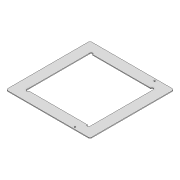
# Autodesk Inventor part: Limiter
Saved by Autodesk Inventor 2020 (Build 240168000, 168)
## iProperties
Created: 2022-04-24
Part Number: Limiter
Material: Generic
Document SubType Name: Modeling
Designer: ferrerx
Density: 1 g/cm^3
Appearance: Default
Author: ferrerx
Autodesk Inventor part; units mm, degrees
ref_plane "YZ Plane" through (0, 0, 0) normal (1, 0, 0) x (0, 1, 0)
ref_plane "XZ Plane" through (0, 0, 0) normal (0, 1, 0) x (-1, 0, 0)
ref_plane "XY Plane" through (0, 0, 0) normal (0, 0, 1) x (1, 0, 0)
sketch "Sketch1" plane through (0, 0, 0) normal (0, 1, 0) x (-1, 0, 0)
  line L0 (-85, 85) -> (85, 85)
  line L1 (85, 85) -> (85, -85)
  line L2 (85, -85) -> (-85, -85)
  line L3 (-85, -85) -> (-85, 85)
  line L4 (-85, 85) -> (85, -85) construction
  line L5 (85, 85) -> (-85, -85) construction
  line L6 (-112.5, 112.5) -> (112.5, 112.5)
  line L7 (112.5, 112.5) -> (112.5, -112.5)
  line L8 (112.5, -112.5) -> (-112.5, -112.5)
  line L9 (-112.5, -112.5) -> (-112.5, 112.5)
  line L10 (-112.5, 112.5) -> (112.5, -112.5) construction
  line L11 (112.5, 112.5) -> (-112.5, -112.5) construction
  point P0 (0, 0)
  dimension "d0" = 170
  dimension "d1" = 170
  dimension "d2" = 225
  dimension "d3" = 225
  constraints: 24 end point, 4 midpoint, 4 parallel, 2 horizontal, 2 perpendicular
  measures "d0" distance of L1.end L2.end
  measures "d1" distance of L2.end L0.start
  measures "d2" distance of L8.end L6.start
  measures "d3" distance of L6.start L6.end
extrude "Extrusion1" add sketch "Sketch1" along normal blind 2
sketch "Sketch2" plane through (0, 2, 0) normal (0, 1, 0) x (1, 0, 0)
  line L0 (0, 0) -> (-112.5, 0) construction
  line L1 (-112.5, 112.5) -> (-112.5, -112.5) projected
  circle A0 centre (66.4, -106.5) radius 1.9
  circle A1 centre (66.4, 106.5) radius 1.9
  dimension "d6" = 66.4
  dimension "d7" = 3.8
  dimension "d8" = 106.5
  constraints: 2 centre point, 2 end point, 1 midpoint, 1 symmetric about line, 1 other
  measures "d6" horizontal distance of L0.start A0.centre
  measures "d7" diameter of A0
  measures "d8" vertical distance of L0.start A0.centre
extrude "Extrusion2" cut sketch "Sketch2" against normal blind 2
fillet "Fillet1" radius 5 4 edges at (112.5, 1, -112.5) (112.5, 1, 112.5) (-112.5, 1, -112.5) (-112.5, 1, 112.5)
sketch "Sketch3" plane through (0, 2, 0) normal (0, 1, 0) x (1, 0, 0)
  line L0 (85, 85) -> (85, -85) projected
  circle A0 centre (81.5, -85) radius 3.5
  line L1 (-85, -85) -> (-85, 85) projected
  line L2 (0, 0) -> (-85, 0) construction
  line L3 (0, 0) -> (0, -85) construction
  line L4 (85, -85) -> (-85, -85) projected
  circle A1 centre (-81.5, -85) radius 3.5
  circle A2 centre (81.5, 85) radius 3.5
  circle A3 centre (-81.5, 85) radius 3.5
  point P0 (-85, -85)
  point P1 (-78, -85)
  dimension "d12" = 7
  constraints: 4 centre point, 4 end point, 3 symmetric about line, 2 midpoint, 1 tangent, 3 other
  measures "d12" diameter of A0
extrude "Extrusion3" cut sketch "Sketch3" against normal blind 2 contours L4 A0 | A0 L4 | A1 L4 | A2 | A3 picked at (-80.4331, -85.8214)
body "Solid1"
